Autodesk Fusion 360 part; units mm, degrees
(part 2 of 2)
  spline S18 degree 5 poles (-7.2517, 9.4747) (-7.3168, 9.512) (-7.4501, 9.5899) (-7.66, 9.7166) (-7.9595, 9.9067) (-8.358, 10.1768) (-8.767, 10.4716) (-9.1708, 10.7803) (-9.5541, 11.0901) (-9.9048, 11.3876) (-10.2171, 11.6603) (-10.4929, 11.8976) (-10.7391, 12.0922) (-10.9658, 12.2407) (-11.1836, 12.3449) (-11.4019, 12.4133) (-11.6267, 12.4594) (-11.861, 12.4958) (-12.1043, 12.5285) (-12.3522, 12.5507) (-12.5988, 12.5473) (-12.8401, 12.5021) (-13.0767, 12.404) (-13.3168, 12.2526) (-13.5718, 12.0543) (-13.8538, 11.8189) (-14.1722, 11.5576) (-14.5304, 11.2787) (-14.9249, 10.987) (-15.3481, 10.6852) (-15.7889, 10.3744) (-16.2353, 10.0552) (-16.6753, 9.7283) (-17.0991, 9.3955) (-17.5005, 9.0606) (-17.8781, 8.73) (-18.2334, 8.4108) (-18.5695, 8.11) (-18.8894, 7.8327) (-19.1946, 7.5816) (-19.4837, 7.3549) (-19.7507, 7.1453) (-19.9856, 6.9408) (-20.1783, 6.7275) (-20.3206, 6.4921) (-20.41, 6.2244) (-20.4512, 5.9192) (-20.4542, 5.5754) (-20.432, 5.194) (-20.3978, 4.777) (-20.3627, 4.3258) (-20.3339, 3.8398) (-20.3149, 3.3177) (-20.3063, 2.7575) (-20.3067, 2.1576) (-20.3131, 1.5176) (-20.3215, 0.8388) (-20.3279, 0.1251) (-20.3285, -0.6164) (-20.3207, -1.3746) (-20.3034, -2.1349) (-20.2759, -2.8807) (-20.239, -3.5949) (-20.1938, -4.2607) (-20.1419, -4.8634) (-20.0857, -5.3913) (-20.0274, -5.8373) (-19.9695, -6.1998) (-19.9146, -6.4846) (-19.8639, -6.7043) (-19.814, -6.8757) (-19.7546, -7.0182) (-19.6644, -7.1514) (-19.5198, -7.2925) (-19.3074, -7.4536) (-19.0351, -7.6386) (-18.7247, -7.8455) (-18.4043, -8.0673) (-18.1006, -8.2943) (-17.8313, -8.5156) (-17.5973, -8.7207) (-17.3875, -8.9016) (-17.1846, -9.0544) (-16.9699, -9.1809) (-16.7295, -9.2913) (-16.4555, -9.402) (-16.1448, -9.531) (-15.7988, -9.6939) (-15.4216, -9.8999) (-15.0203, -10.1472) (-14.604, -10.4266) (-14.1834, -10.7236) (-13.7708, -11.0211) (-13.3794, -11.3028) (-13.023, -11.5549) (-12.7157, -11.7699) (-12.4712, -11.9479) (-12.2956, -12.0935) (-12.1833, -12.2134) (-12.1094, -12.313) (-12.0269, -12.3943) (-11.8938, -12.4605) (-11.7016, -12.5203) (-11.4667, -12.5825) (-11.2156, -12.6491) (-10.971, -12.7069) (-10.7469, -12.7327) (-10.5487, -12.7034) (-10.3698, -12.6053) (-10.1927, -12.4403) (-9.9959, -12.2196) (-9.76, -11.9595) (-9.4757, -11.6758) (-9.1465, -11.3808) (-8.7837, -11.084) (-8.4031, -10.7925) (-8.0218, -10.5104) (-7.6537, -10.2396) (-7.3069, -9.9797) (-6.9789, -9.7282) (-6.6609, -9.4812) (-6.3406, -9.2345) (-6.0056, -8.9846) (-5.6472, -8.7296) (-5.2637, -8.4697) (-4.8637, -8.2089) (-4.4636, -7.9529) (-4.0833, -7.7077) (-3.743, -7.4773) (-3.4589, -7.2624) (-3.2401, -7.0583) (-3.084, -6.8528) (-2.9785, -6.6295) (-2.9084, -6.3746) (-2.8592, -6.0822) (-2.8238, -5.7618) (-2.801, -5.4333) (-2.7922, -5.1182) (-2.7991, -4.8328) (-2.8206, -4.5793) (-2.8513, -4.3413) (-2.8836, -4.0939) (-2.9103, -3.8111) (-2.9266, -3.4759) (-2.9318, -3.0849) (-2.9277, -2.6437) (-2.9179, -2.1642) (-2.9066, -1.6617) (-2.898, -1.1512) (-2.8953, -0.6444) (-2.8997, -0.1471) (-2.9108, 0.3397) (-2.9278, 0.8181) (-2.9493, 1.2924) (-2.9742, 1.7676) (-3.0021, 2.2478) (-3.0339, 2.7355) (-3.0722, 3.2296) (-3.12, 3.7267) (-3.1797, 4.2204) (-3.2516, 4.7025) (-3.3331, 5.1626) (-3.4174, 5.5887) (-3.4923, 5.9676) (-3.54, 6.2851) (-3.5462, 6.5321) (-3.5083, 6.7085) (-3.4435, 6.8282) (-3.397, 6.9241) (-3.4176, 7.0322) (-3.5281, 7.1723) (-3.7286, 7.3497) (-4.0048, 7.5599) (-4.3366, 7.7927) (-4.7008, 8.035) (-5.0747, 8.2729) (-5.4384, 8.494) (-5.7777, 8.6901) (-6.0873, 8.859) (-6.3735, 9.0076) (-6.6504, 9.1484) (-6.8781, 9.2669) (-7.0596, 9.3657) (-7.1866, 9.4373) (-7.2517, 9.4747) knots 0 0 0 0 0 0 0.00555556 0.01111111 0.01666667 0.02222222 0.02777778 0.03333333 0.03888889 0.04444444 0.05 0.05555556 0.06111111 0.06666667 0.07222222 0.07777778 0.08333333 0.08888889 0.09444444 0.1 0.10555556 0.11111111 0.11666667 0.12222222 0.12777778 0.13333333 0.13888889 0.14444444 0.15 0.15555556 0.16111111 0.16666667 0.17222222 0.17777778 0.18333333 0.18888889 0.19444444 0.2 0.20555556 0.21111111 0.21666667 0.22222222 0.22777778 0.23333333 0.23888889 0.24444444 0.25 0.25555556 0.26111111 0.26666667 0.27222222 0.27777778 0.28333333 0.28888889 0.29444444 0.3 0.30555556 0.31111111 0.31666667 0.32222222 0.32777778 0.33333333 0.33888889 0.34444444 0.35 0.35555556 0.36111111 0.36666667 0.37222222 0.37777778 0.38333333 0.38888889 0.39444444 0.4 0.40555556 0.41111111 0.41666667 0.42222222 0.42777778 0.43333333 0.43888889 0.44444444 0.45 0.45555556 0.46111111 0.46666667 0.47222222 0.47777778 0.48333333 0.48888889 0.49444444 0.5 0.50555556 0.51111111 0.51666667 0.52222222 0.52777778 0.53333333 0.53888889 0.54444444 0.55 0.55555556 0.56111111 0.56666667 0.57222222 0.57777778 0.58333333 0.58888889 0.59444444 0.6 0.60555556 0.61111111 0.61666667 0.62222222 0.62777778 0.63333333 0.63888889 0.64444444 0.65 0.65555556 0.66111111 0.66666667 0.67222222 0.67777778 0.68333333 0.68888889 0.69444444 0.7 0.70555556 0.71111111 0.71666667 0.72222222 0.72777778 0.73333333 0.73888889 0.74444444 0.75 0.75555556 0.76111111 0.76666667 0.77222222 0.77777778 0.78333333 0.78888889 0.79444444 0.8 0.80555556 0.81111111 0.81666667 0.82222222 0.82777778 0.83333333 0.83888889 0.84444444 0.85 0.85555556 0.86111111 0.86666667 0.87222222 0.87777778 0.88333333 0.88888889 0.89444444 0.9 0.90555556 0.91111111 0.91666667 0.92222222 0.92777778 0.93333333 0.93888889 0.94444444 0.95 0.95555556 0.96111111 0.96666667 0.97222222 0.97777778 0.98333333 0.98888889 0.99444444 1 1 1 1 1 1
  spline S19 degree 5 poles (-40.2, 19.4351) (-40.1495, 19.476) (-40.0504, 19.5572) (-39.9066, 19.6793) (-39.7159, 19.8475) (-39.453, 20.0809) (-39.14, 20.3488) (-38.758, 20.6585) (-38.3003, 21.011) (-37.7793, 21.3986) (-37.2214, 21.8068) (-36.6606, 22.217) (-36.1323, 22.6084) (-35.6682, 22.9604) (-35.2892, 23.2551) (-35.0009, 23.4794) (-34.785, 23.6273) (-34.6008, 23.7015) (-34.4066, 23.7119) (-34.1775, 23.6741) (-33.9251, 23.6084) (-33.6789, 23.5323) (-33.471, 23.4545) (-33.3152, 23.365) (-33.2061, 23.2403) (-33.1308, 23.057) (-33.0779, 22.8053) (-33.0386, 22.4862) (-33.0065, 22.1076) (-32.977, 21.6793) (-32.9478, 21.209) (-32.9178, 20.7018) (-32.8874, 20.1618) (-32.8573, 19.593) (-32.8288, 19.0006) (-32.8028, 18.3916) (-32.7799, 17.7766) (-32.7595, 17.1703) (-32.7405, 16.59) (-32.7226, 16.0527) (-32.7068, 15.5729) (-32.6961, 15.1596) (-32.6968, 14.8144) (-32.7192, 14.5282) (-32.7779, 14.2806) (-32.8886, 14.0459) (-33.0655, 13.7986) (-33.3183, 13.5197) (-33.6503, 13.1997) (-34.0603, 12.8358) (-34.5422, 12.4316) (-35.0857, 11.9949) (-35.6774, 11.5367) (-36.3007, 11.0697) (-36.9368, 10.6072) (-37.5651, 10.161) (-38.1648, 9.7421) (-38.7171, 9.3602) (-39.207, 9.0239) (-39.6256, 8.7411) (-39.9715, 8.5185) (-40.2533, 8.362) (-40.4915, 8.2769) (-40.7195, 8.2675) (-40.9724, 8.3353) (-41.2796, 8.4772) (-41.6523, 8.6835) (-42.0841, 8.9384) (-42.5573, 9.2226) (-43.047, 9.5149) (-43.5268, 9.7948) (-43.9737, 10.0443) (-44.373, 10.25) (-44.7229, 10.4053) (-45.0277, 10.511) (-45.2924, 10.5774) (-45.5183, 10.6236) (-45.6944, 10.6818) (-45.8041, 10.7888) (-45.8443, 10.969) (-45.8452, 11.2162) (-45.854, 11.5036) (-45.9111, 11.7986) (-46.0261, 12.078) (-46.1667, 12.3364) (-46.2851, 12.578) (-46.3335, 12.8126) (-46.2887, 13.0483) (-46.157, 13.2899) (-45.9588, 13.5405) (-45.7197, 13.8029) (-45.4577, 14.0807) (-45.1827, 14.3782) (-44.899, 14.6991) (-44.6065, 15.0456) (-44.3031, 15.4178) (-43.9864, 15.8126) (-43.6548, 16.2231) (-43.3079, 16.6403) (-42.9465, 17.0538) (-42.5731, 17.4534) (-42.1923, 17.8296) (-41.8102, 18.1754) (-41.4361, 18.4869) (-41.0804, 18.7639) (-40.7523, 19.0098) (-40.5162, 19.1867) (-40.3537, 19.3122) (-40.2505, 19.3943) (-40.2, 19.4351) knots 0 0 0 0 0 0 0.00952381 0.01904762 0.02857143 0.03809524 0.04761905 0.05714286 0.06666667 0.07619048 0.08571429 0.0952381 0.1047619 0.11428571 0.12380952 0.13333333 0.14285714 0.15238095 0.16190476 0.17142857 0.18095238 0.19047619 0.2 0.20952381 0.21904762 0.22857143 0.23809524 0.24761905 0.25714286 0.26666667 0.27619048 0.28571429 0.2952381 0.3047619 0.31428571 0.32380952 0.33333333 0.34285714 0.35238095 0.36190476 0.37142857 0.38095238 0.39047619 0.4 0.40952381 0.41904762 0.42857143 0.43809524 0.44761905 0.45714286 0.46666667 0.47619048 0.48571429 0.4952381 0.5047619 0.51428571 0.52380952 0.53333333 0.54285714 0.55238095 0.56190476 0.57142857 0.58095238 0.59047619 0.6 0.60952381 0.61904762 0.62857143 0.63809524 0.64761905 0.65714286 0.66666667 0.67619048 0.68571429 0.6952381 0.7047619 0.71428571 0.72380952 0.73333333 0.74285714 0.75238095 0.76190476 0.77142857 0.78095238 0.79047619 0.8 0.80952381 0.81904762 0.82857143 0.83809524 0.84761905 0.85714286 0.86666667 0.87619048 0.88571429 0.8952381 0.9047619 0.91428571 0.92380952 0.93333333 0.94285714 0.95238095 0.96190476 0.97142857 0.98095238 0.99047619 1 1 1 1 1 1
  spline S20 degree 5 poles (-25.9, 8.6722) (-25.985, 8.7472) (-26.1636, 8.9038) (-26.4606, 9.1593) (-26.9174, 9.5357) (-27.5668, 10.0317) (-28.2524, 10.5092) (-28.9256, 10.925) (-29.5423, 11.2473) (-30.0755, 11.4668) (-30.5261, 11.6065) (-30.9112, 11.7) (-31.2555, 11.7738) (-31.5798, 11.825) (-31.895, 11.8119) (-32.2111, 11.6854) (-32.5455, 11.4204) (-32.9254, 11.0283) (-33.3782, 10.5415) (-33.9245, 10.003) (-34.5714, 9.4557) (-35.3028, 8.9294) (-36.0811, 8.4376) (-36.8574, 7.9821) (-37.5787, 7.5557) (-38.1966, 7.1453) (-38.6754, 6.7349) (-39.0006, 6.3087) (-39.1866, 5.8539) (-39.2658, 5.3609) (-39.2789, 4.8233) (-39.2645, 4.2377) (-39.2483, 3.604) (-39.2441, 2.9246) (-39.2565, 2.2046) (-39.2832, 1.4506) (-39.3166, 0.6707) (-39.3466, -0.1262) (-39.3626, -0.9307) (-39.3551, -1.7331) (-39.3175, -2.5235) (-39.2478, -3.2923) (-39.1505, -4.0305) (-39.0386, -4.7293) (-38.934, -5.3811) (-38.859, -5.9806) (-38.8263, -6.5264) (-38.8314, -7.0222) (-38.8419, -7.4784) (-38.7927, -7.9128) (-38.6115, -8.3453) (-38.2383, -8.7928) (-37.6502, -9.2644) (-36.8736, -9.7584) (-35.9659, -10.2657) (-35.0038, -10.7727) (-34.0691, -11.2633) (-33.2357, -11.7224) (-32.5556, -12.138) (-32.0455, -12.504) (-31.6741, -12.823) (-31.3816, -13.0981) (-31.0981, -13.3257) (-30.7625, -13.488) (-30.3407, -13.5461) (-29.8195, -13.456) (-29.202, -13.1834) (-28.5022, -12.7205) (-27.7405, -12.0969) (-26.9418, -11.3666) (-26.1335, -10.5978) (-25.3437, -9.8614) (-24.599, -9.2207) (-23.9227, -8.7192) (-23.3325, -8.3717) (-22.8388, -8.1491) (-22.4442, -7.9856) (-22.1471, -7.8007) (-21.9423, -7.5148) (-21.8245, -7.0705) (-21.7873, -6.4359) (-21.8233, -5.6001) (-21.9228, -4.5723) (-22.0736, -3.3784) (-22.26, -2.0594) (-22.4625, -0.6688) (-22.6569, 0.7295) (-22.8183, 2.0679) (-22.9253, 3.2821) (-22.9644, 4.3176) (-22.9339, 5.137) (-22.8485, 5.7265) (-22.743, 6.1028) (-22.6769, 6.3201) (-22.7387, 6.4772) (-22.9915, 6.6663) (-23.409, 6.9138) (-23.9101, 7.2016) (-24.4022, 7.495) (-24.8205, 7.7682) (-25.1705, 8.0316) (-25.4353, 8.2591) (-25.6538, 8.454) (-25.815, 8.5972) (-25.9, 8.6722) knots 0 0 0 0 0 0 0.01 0.02 0.03 0.04 0.05 0.06 0.07 0.08 0.09 0.1 0.11 0.12 0.13 0.14 0.15 0.16 0.17 0.18 0.19 0.2 0.21 0.22 0.23 0.24 0.25 0.26 0.27 0.28 0.29 0.3 0.31 0.32 0.33 0.34 0.35 0.36 0.37 0.38 0.39 0.4 0.41 0.42 0.43 0.44 0.45 0.46 0.47 0.48 0.49 0.5 0.51 0.52 0.53 0.54 0.55 0.56 0.57 0.58 0.59 0.6 0.61 0.62 0.63 0.64 0.65 0.66 0.67 0.68 0.69 0.7 0.71 0.72 0.73 0.74 0.75 0.76 0.77 0.78 0.79 0.8 0.81 0.82 0.83 0.84 0.85 0.86 0.87 0.88 0.89 0.9 0.91 0.92 0.93 0.94 0.95 0.96 0.97 0.98 0.99 1 1 1 1 1 1
  spline S21 degree 5 poles (-40.2, -20.1) (-40.0706, -20.2092) (-39.8095, -20.4267) (-39.4106, -20.7506) (-38.8646, -21.1776) (-38.1588, -21.703) (-37.4319, -22.2187) (-36.6888, -22.7225) (-35.9379, -23.2109) (-35.1929, -23.6784) (-34.4731, -24.1178) (-33.8055, -24.5194) (-33.2254, -24.8707) (-32.767, -25.1588) (-32.4534, -25.373) (-32.2867, -25.5066) (-32.2382, -25.5597) (-32.2349, -25.5425) (-32.1855, -25.4699) (-32.0198, -25.3543) (-31.7004, -25.2031) (-31.3079, -25.0569) (-30.9345, -24.9337) (-30.6507, -24.8456) (-30.5, -24.8) knots 0 0 0 0 0 0 0.05 0.1 0.15 0.2 0.25 0.3 0.35 0.4 0.45 0.5 0.55 0.6 0.65 0.7 0.75 0.8 0.85 0.9 0.95 1 1 1 1 1 1
  spline S22 degree 5 poles (-30.5, -24.8) (-30.4964, -24.8106) (-30.4893, -24.8249) (-30.4795, -24.8259) (-30.4679, -24.7865) (-30.4563, -24.6722) (-30.4484, -24.5015) (-30.4456, -24.2861) (-30.4488, -24.0388) (-30.4584, -23.7715) (-30.4736, -23.4928) (-30.4933, -23.2086) (-30.5154, -22.9229) (-30.538, -22.6377) (-30.5591, -22.3537) (-30.5769, -22.0706) (-30.5902, -21.7877) (-30.5984, -21.5037) (-30.6017, -21.2168) (-30.6011, -20.925) (-30.5987, -20.6258) (-30.5975, -20.317) (-30.6016, -19.9961) (-30.6152, -19.6614) (-30.6417, -19.3126) (-30.6835, -18.9504) (-30.7409, -18.5781) (-30.8118, -18.2012) (-30.8907, -17.8283) (-30.97, -17.47) (-31.042, -17.1373) (-31.0999, -16.8407) (-31.1399, -16.5885) (-31.1622, -16.3858) (-31.1736, -16.2329) (-31.1863, -16.1249) (-31.214, -16.0519) (-31.2687, -15.9993) (-31.3575, -15.949) (-31.4842, -15.883) (-31.6493, -15.7887) (-31.8513, -15.6612) (-32.0873, -15.5007) (-32.3533, -15.3116) (-32.6447, -15.1001) (-32.9573, -14.8733) (-33.2878, -14.6368) (-33.6334, -14.3946) (-33.992, -14.1497) (-34.3617, -13.904) (-34.7407, -13.6587) (-35.1266, -13.4147) (-35.5167, -13.1729) (-35.9073, -12.9341) (-36.2936, -12.6997) (-36.6695, -12.4717) (-37.0284, -12.2525) (-37.3639, -12.0448) (-37.6698, -11.8513) (-37.9417, -11.6746) (-38.1766, -11.517) (-38.3742, -11.3804) (-38.537, -11.2662) (-38.6707, -11.1747) (-38.7834, -11.1053) (-38.8853, -11.0562) (-38.9886, -11.0241) (-39.1062, -11.0048) (-39.2492, -10.9943) (-39.4255, -10.9898) (-39.6398, -10.9896) (-39.8434, -10.9922) (-40.0145, -10.9955) (-40.1368, -10.9984) (-40.2, -11) knots 0 0 0 0 0 0 0.01428571 0.02857143 0.04285714 0.05714286 0.07142857 0.08571429 0.1 0.11428571 0.12857143 0.14285714 0.15714286 0.17142857 0.18571429 0.2 0.21428571 0.22857143 0.24285714 0.25714286 0.27142857 0.28571429 0.3 0.31428571 0.32857143 0.34285714 0.35714286 0.37142857 0.38571429 0.4 0.41428571 0.42857143 0.44285714 0.45714286 0.47142857 0.48571429 0.5 0.51428571 0.52857143 0.54285714 0.55714286 0.57142857 0.58571429 0.6 0.61428571 0.62857143 0.64285714 0.65714286 0.67142857 0.68571429 0.7 0.71428571 0.72857143 0.74285714 0.75714286 0.77142857 0.78571429 0.8 0.81428571 0.82857143 0.84285714 0.85714286 0.87142857 0.88571429 0.9 0.91428571 0.92857143 0.94285714 0.95714286 0.97142857 0.98571429 1 1 1 1 1 1
  spline S23 degree 5 poles (-11.3807, -26) (-11.3882, -25.9105) (-11.4027, -25.7292) (-11.4225, -25.45) (-11.4453, -25.0635) (-11.4676, -24.5565) (-11.484, -24.0265) (-11.4948, -23.4746) (-11.5006, -22.903) (-11.5022, -22.315) (-11.501, -21.7149) (-11.4985, -21.1088) (-11.4968, -20.5044) (-11.4986, -19.911) (-11.506, -19.3381) (-11.5212, -18.7953) (-11.5452, -18.2908) (-11.5783, -17.8313) (-11.619, -17.4208) (-11.6644, -17.0598) (-11.7089, -16.7448) (-11.7463, -16.4683) (-11.7735, -16.2221) (-11.7943, -15.999) (-11.8223, -15.795) (-11.8853, -15.6121) (-12.009, -15.4539) (-12.2023, -15.3221) (-12.4367, -15.2119) (-12.6554, -15.113) (-12.8073, -15.0148) (-12.8724, -14.9108) (-12.8948, -14.8037) (-12.9486, -14.6996) (-13.0853, -14.5989) (-13.3163, -14.4937) (-13.6305, -14.3727) (-14.0028, -14.2244) (-14.4069, -14.0412) (-14.8248, -13.8219) (-15.2451, -13.5706) (-15.6619, -13.2949) (-16.0729, -13.0046) (-16.4785, -12.71) (-16.8799, -12.4202) (-17.2784, -12.1423) (-17.6731, -11.879) (-18.0611, -11.629) (-18.4373, -11.3894) (-18.7951, -11.1568) (-19.1266, -10.9294) (-19.4222, -10.7085) (-19.6719, -10.4999) (-19.8642, -10.3165) (-19.9921, -10.1728) (-20.0597, -10.0773) (-20.0887, -10.0256) (-20.1237, -9.9948) (-20.2069, -9.9655) (-20.3606, -9.9346) (-20.5879, -9.9046) (-20.8677, -9.8779) (-21.1654, -9.856) (-21.4457, -9.842) (-21.6827, -9.8418) (-21.8755, -9.8663) (-22.048, -9.9302) (-22.2323, -10.0471) (-22.4581, -10.2255) (-22.7378, -10.4644) (-23.0703, -10.7553) (-23.4448, -11.0849) (-23.8443, -11.4371) (-24.2493, -11.7957) (-24.642, -12.1464) (-25.0092, -12.4795) (-25.3469, -12.7922) (-25.6587, -13.0874) (-25.9525, -13.3714) (-26.2386, -13.6516) (-26.5268, -13.9345) (-26.8236, -14.2239) (-27.1301, -14.5183) (-27.4395, -14.8093) (-27.7397, -15.0856) (-28.0164, -15.336) (-28.2555, -15.5537) (-28.4458, -15.7392) (-28.5816, -15.9048) (-28.6652, -16.076) (-28.7033, -16.2816) (-28.7055, -16.5469) (-28.6814, -16.8826) (-28.6397, -17.2845) (-28.5884, -17.7384) (-28.5342, -18.2242) (-28.483, -18.7198) (-28.4394, -19.2053) (-28.4066, -19.6669) (-28.3867, -20.1014) (-28.3802, -20.5139) (-28.3864, -20.9144) (-28.4038, -21.3151) (-28.4297, -21.727) (-28.4606, -22.1572) (-28.4923, -22.6051) (-28.5201, -23.0611) (-28.5393, -23.5103) (-28.5459, -23.9357) (-28.5369, -24.3208) (-28.511, -24.6538) (-28.4693, -24.9298) (-28.4156, -25.1551) (-28.3556, -25.3436) (-28.2954, -25.5118) (-28.2397, -25.6733) (-28.2007, -25.8027) (-28.1749, -25.9009) (-28.1593, -25.9669) (-28.1519, -26) knots 0 0 0 0 0 0 0.00869565 0.0173913 0.02608696 0.03478261 0.04347826 0.05217391 0.06086957 0.06956522 0.07826087 0.08695652 0.09565217 0.10434783 0.11304348 0.12173913 0.13043478 0.13913043 0.14782609 0.15652174 0.16521739 0.17391304 0.1826087 0.19130435 0.2 0.20869565 0.2173913 0.22608696 0.23478261 0.24347826 0.25217391 0.26086957 0.26956522 0.27826087 0.28695652 0.29565217 0.30434783 0.31304348 0.32173913 0.33043478 0.33913043 0.34782609 0.35652174 0.36521739 0.37391304 0.3826087 0.39130435 0.4 0.40869565 0.4173913 0.42608696 0.43478261 0.44347826 0.45217391 0.46086957 0.46956522 0.47826087 0.48695652 0.49565217 0.50434783 0.51304348 0.52173913 0.53043478 0.53913043 0.54782609 0.55652174 0.56521739 0.57391304 0.5826087 0.59130435 0.6 0.60869565 0.6173913 0.62608696 0.63478261 0.64347826 0.65217391 0.66086957 0.66956522 0.67826087 0.68695652 0.69565217 0.70434783 0.71304348 0.72173913 0.73043478 0.73913043 0.74782609 0.75652174 0.76521739 0.77391304 0.7826087 0.79130435 0.8 0.80869565 0.8173913 0.82608696 0.83478261 0.84347826 0.85217391 0.86086957 0.86956522 0.87826087 0.88695652 0.89565217 0.90434783 0.91304348 0.92173913 0.93043478 0.93913043 0.94782609 0.95652174 0.96521739 0.97391304 0.9826087 0.99130435 1 1 1 1 1 1
  spline S24 degree 5 poles (-35.5, -26) (-35.5833, -25.9533) (-35.751, -25.8583) (-36.0053, -25.7111) (-36.3502, -25.5056) (-36.7917, -25.2319) (-37.2442, -24.9401) (-37.7088, -24.629) (-38.1855, -24.2981) (-38.6736, -23.9487) (-39.1723, -23.5822) (-39.5789, -23.2765) (-39.8879, -23.0408) (-40.0957, -22.8807) (-40.2, -22.8) knots 0 0 0 0 0 0 0.1 0.2 0.3 0.4 0.5 0.6 0.7 0.8 0.9 1 1 1 1 1 1
  spline S25 degree 5 poles (14.0457, 25.2) (14.0267, 25.2099) (13.9912, 25.2275) (13.9457, 25.2475) (13.8992, 25.2627) (13.862, 25.2643) (13.8508, 25.2507) (13.8556, 25.2299) (13.8653, 25.2109) (13.8718, 25.2) knots 0 0 0 0 0 0 0.2 0.4 0.6 0.8 1 1 1 1 1 1
  line L8 (14.1082, 25.1676) -> (13.9832, 25.2324)
  line L9 (13.8589, 25.2215) -> (13.8846, 25.1785)
  spline S26 degree 5 poles (21.4, 18.8332) (21.4048, 18.832) (21.414, 18.8302) (21.426, 18.8289) (21.4384, 18.8303) (21.4449, 18.8396) (21.4384, 18.8571) (21.4237, 18.8786) (21.4087, 18.8973) (21.4, 18.9077) knots 0 0 0 0 0 0 0.2 0.4 0.6 0.8 1 1 1 1 1 1
  line L10 (21.44, 18.8599) -> (21.36, 18.9555)
  spline S27 degree 5 poles (21.4, 18.75) (21.3631, 18.7928) (21.2889, 18.8779) (21.1763, 19.0041) (21.0237, 19.1697) (20.829, 19.3722) (20.6305, 19.5711) (20.4291, 19.7678) (20.2261, 19.9649) (20.0229, 20.1657) (19.82, 20.3737) (19.6162, 20.5922) (19.408, 20.8236) (19.1896, 21.0695) (18.9547, 21.3303) (18.6977, 21.6059) (18.4144, 21.8949) (18.1039, 22.1949) (17.7674, 22.5031) (17.4075, 22.8161) (17.0278, 23.1307) (16.6321, 23.4439) (16.2236, 23.7531) (15.8046, 24.0568) (15.3767, 24.3539) (14.9409, 24.6439) (14.5864, 24.87) (14.3173, 25.0363) (14.1365, 25.1457) (14.0457, 25.2) knots 0 0 0 0 0 0 0.04 0.08 0.12 0.16 0.2 0.24 0.28 0.32 0.36 0.4 0.44 0.48 0.52 0.56 0.6 0.64 0.68 0.72 0.76 0.8 0.84 0.88 0.92 0.96 1 1 1 1 1 1
  line L11 (-40.2, -0.0059) -> (-9.4, -0.0059) construction
  line L12 (-9.4, -0.0059) -> (4.6, -0.0059) construction
  line L13 (-9.4, -0.0059) -> (-23.4, -0.0059) construction
  line L14 (4.6, -0.0059) -> (4.6, -6.0059) construction
  line L15 (-23.4, -0.0059) -> (-23.4, 5.9941) construction
  line L16 (19.4, -22) -> (19.4, 21.2)
  line L17 (17.4, 23.2) -> (-36.2, 23.2)
  line L18 (-38.2, 21.2) -> (-38.2, -22)
  line L19 (-36.2, -24) -> (17.4, -24)
  arc A23 (17.4, -24) -> (19.4, -22) centre (17.4, -22) ccw
  arc A24 (19.4, 21.2) -> (17.4, 23.2) centre (17.4, 21.2) ccw
  arc A25 (-36.2, 23.2) -> (-38.2, 21.2) centre (-36.2, 21.2) ccw
  arc A26 (-38.2, -22) -> (-36.2, -24) centre (-36.2, -22) ccw
  line L20 (4.6, -6.0059) -> (4.6, -8.2559)
  line L21 (-21.475, 9.1404) -> (2.675, 9.1404)
  line L22 (2.675, 9.1404) -> (2.675, -9.1523)
  line L23 (2.675, -9.1523) -> (-21.475, -9.1523)
  line L24 (-21.475, -9.1523) -> (-21.475, 9.1404)
  line L25 (-21.475, 9.1404) -> (2.675, -9.1523) construction
  line L26 (2.675, 9.1404) -> (-21.475, -9.1523) construction
  line L27 (-22.475, 10.1404) -> (3.675, 10.1404)
  line L28 (3.675, 10.1404) -> (3.675, -10.1523)
  line L29 (3.675, -10.1523) -> (-22.475, -10.1523)
  line L30 (-22.475, -10.1523) -> (-22.475, 10.1404)
  line L31 (2.675, 9.1404) -> (-21.475, 9.1404) construction
  line L32 (-21.475, 9.1404) -> (-21.475, -8.6556) construction
  line L33 (-21.475, -8.6556) -> (2.675, -8.6556) construction
  line L34 (2.675, -8.6556) -> (2.675, 9.1404) construction
  point P0 (7.051, -15.0762)
  point P1 (6.8334, -14.8314)
  point P2 (5.8, -14)
  point P3 (5.004, -13.2468)
  point P4 (3, -11.9)
  point P5 (2.1938, -11.2552)
  point P6 (0.6849, -10.1414)
  point P7 (-0.5285, -9.419)
  point P8 (-1.3037, -9.3762)
  point P9 (-2.3649, -9.4289)
  point P10 (-2.8331, -9.5374)
  point P11 (-5.5, -11.6)
  point P12 (-8.6, -14.2)
  point P13 (-9.7727, -15.2896)
  point P14 (-9.8476, -15.4656)
  point P15 (-9.85, -15.9)
  point P16 (-9.9, -19.4)
  point P17 (-9.7, -24)
  point P18 (19.8, -9.5)
  point P19 (18.3, -8.5)
  point P20 (18, -8.4)
  point P21 (16.7, -8.45)
  point P22 (16.2684, -8.4722)
  point P23 (16.0731, -8.5685)
  point P24 (13.8, -10.4)
  point P25 (10.9, -12.8)
  point P26 (9.4, -14.3)
  point P27 (19.1566, -6.6508)
  point P28 (18.8, -6.4)
  point P29 (18.7, -6.3)
  point P30 (18.55, -5.75)
  point P31 (18.2, -4.9)
  point P32 (18.3, -3.5)
  point P33 (18.5, -1.9)
  point P34 (18.5, 1.2)
  point P35 (18.3, 5.1)
  point P36 (18.3, 6.4)
  point P37 (18.1, 7.7)
  point P38 (18.1, 7.9)
  point P39 (18.9, 8.7)
  point P40 (19.8, 9.4)
  point P41 (13.5, -6.7)
  point P42 (11.8, -8.2)
  point P43 (11.2358, -8.9708)
  point P44 (9.7, -10.7)
  point P45 (8.9, -11.5)
  point P46 (7.1, -11.8)
  point P47 (6.9515, -11.7173)
  point P48 (6.7172, -11.5441)
  point P49 (6.1776, -11.2025)
  point P50 (5.2568, -10.5309)
  point P51 (3.2, -9)
  point P52 (1.1, -7.7)
  point P53 (-0.3, -6.9)
  point P54 (-0.4238, -6.8342)
  point P55 (-0.5, -6.65)
  point P56 (-1.1, -5.6)
  point P57 (-1.03, -5.44)
  point P58 (-1, -5.06)
  point P59 (-1.2, 0.8)
  point P60 (-1.4, 3.6)
  point P61 (-1.3471, 6.431)
  point P62 (-1.25, 6.6)
  point P63 (-0.95, 7)
  point P64 (0.1, 8.2)
  point P65 (1.3456, 9.4747)
  point P66 (2.8, 10.4)
  point P67 (4.9, 11.6)
  point P68 (6.3872, 12.6401)
  point P69 (6.6424, 12.7645)
  point P70 (6.8339, 12.9272)
  point P71 (6.853, 13.1666)
  point P72 (8.7389, 12.6752)
  point P73 (9.9, 11.8)
  point P74 (11.8532, 10.4191)
  point P75 (14.6, 8.6)
  point P76 (15.0195, 8.3059)
  point P77 (15.3239, 7.4349)
  point P78 (15.4241, 7.0187)
  point P79 (15.46, 6.97)
  point P80 (15.47, 6.82)
  point P81 (15.5, 5.3)
  point P82 (15.7, 1.7)
  point P83 (15.9, -1.6)
  point P84 (16, -4.7)
  point P85 (19, 12.5)
  point P86 (17.1, 10.8)
  point P87 (16.9413, 10.7222)
  point P88 (15.4242, 10.653)
  point P89 (15.2561, 10.5355)
  point P90 (14.7, 10.9)
  point P91 (13, 12.2)
  point P92 (9.9, 14.1)
  point P93 (8.3, 15.2)
  point P94 (8.1, 15.6)
  point P95 (7.6, 16.4)
  point P96 (7.5842, 24.746)
  point P97 (7.7, 25)
  point P98 (11.1, 24.8)
  point P99 (13.2, 23.5)
  point P100 (15.3, 21.9)
  point P101 (19.7684, 17.8233)
  point P102 (-1.7373, 10.1137)
  point P103 (-2, 10)
  point P104 (-3.9745, 10.1787)
  point P105 (-4.5, 10.5)
  point P106 (-8.6013, 13.0644)
  point P107 (-11, 15)
  point P108 (-11.4088, 17.8233)
  point P109 (-11.8416, 24.856)
  point P110 (-11.8416, 28.1549)
  point P111 (5.5887, 19.6873)
  point P112 (-13.7842, 19.4469)
  point P113 (-13.4708, 14.953)
  point P114 (-14.3, 14.3)
  point P115 (-17.1, 12.1)
  point P116 (-20.1, 9.7)
  point P117 (-20.4418, 9.3773)
  point P118 (-20.9233, 9.2608)
  point P119 (-22.6453, 9.1404)
  point P120 (-23.25, 9.6)
  point P121 (-25.9, 11.2)
  point P122 (-27, 12)
  point P123 (-29.5, 13.6)
  point P124 (-29.7216, 13.8493)
  point P125 (-30.059, 14.4103)
  point P126 (-30.2, 14.8)
  point P127 (-30.275, 15.4915)
  point P128 (-30.5, 18)
  point P129 (-30.6157, 22.6489)
  point P130 (-30.3715, 24.2766)
  point P131 (-37.4, 24)
  point P132 (-9.8, 11.3)
  point P133 (-11.1, 12.3)
  point P134 (-11.9, 12.5)
  point P135 (-12.8, 12.5)
  point P136 (-14, 11.7)
  point P137 (-16.9943, 9.4747)
  point P138 (-19.3, 7.5)
  point P139 (-20.3, 6.5)
  point P140 (-20.4, 4.8)
  point P141 (-20.3271, -0.0959)
  point P142 (-20, -6)
  point P143 (-19.8, -6.9)
  point P144 (-19.5, -7.3)
  point P145 (-18.1, -8.3)
  point P146 (-17.1, -9.1)
  point P147 (-15.8, -9.7)
  point P148 (-13.1, -11.5)
  point P149 (-12.2, -12.2)
  point P150 (-12, -12.4)
  point P151 (-11.4, -12.6)
  point P152 (-10.6, -12.7)
  point P153 (-9.8455, -12.0566)
  point P154 (-7.6497, -10.2354)
  point P155 (-5.6, -8.7)
  point P156 (-3.4, -7.2)
  point P157 (-2.9, -6.3)
  point P158 (-2.8, -4.9)
  point P159 (-2.9, -3.9)
  point P160 (-2.9, -1.2)
  point P161 (-3, 2.2)
  point P162 (-3.4, 5.5)
  point P163 (-3.5, 6.7)
  point P164 (-3.4128, 6.9443)
  point P165 (-3.8, 7.4)
  point P166 (-5.8, 8.7)
  point P167 (-38.7, 20.7)
  point P168 (-35.1, 23.4)
  point P169 (-34.4, 23.7)
  point P170 (-33.6, 23.5)
  point P171 (-33.2, 23.2)
  point P172 (-33, 22)
  point P173 (-32.8, 18.3)
  point P174 (-32.7, 14.9)
  point P175 (-33, 13.9)
  point P176 (-36.4, 11)
  point P177 (-40.2, 8.4)
  point P178 (-41.1, 8.4)
  point P179 (-43.9, 10)
  point P180 (-45.4, 10.6)
  point P181 (-45.7987, 10.8317)
  point P182 (-45.9, 11.7)
  point P183 (-46.3, 12.7)
  point P184 (-45.9, 13.6)
  point P185 (-44.4, 15.3)
  point P186 (-42, 18)
  point P187 (-29.4758, 11.2)
  point P188 (-31.171, 11.7528)
  point P189 (-32.0838, 11.7202)
  point P190 (-34.2191, 9.7643)
  point P191 (-38.62, 6.7488)
  point P192 (-39.272, 4.744)
  point P193 (-39.3046, 0.9461)
  point P194 (-39.1579, -3.9438)
  point P195 (-38.8319, -6.9266)
  point P196 (-38.3266, -8.6544)
  point P197 (-32.6217, -12.11)
  point P198 (-31.1, -13.3)
  point P199 (-29.3, -13.2)
  point P200 (-23.7, -8.6)
  point P201 (-22.1, -7.7)
  point P202 (-22.2711, -1.9916)
  point P203 (-22.7504, 6.0736)
  point P204 (-22.8, 6.5)
  point P205 (-24.4, 7.5)
  point P206 (-34.5, -24.1)
  point P207 (-32.3, -25.5)
  point P208 (-32.2, -25.5)
  point P209 (-30.4701, -24.7787)
  point P210 (-30.45, -24.05)
  point P211 (-30.5507, -22.4626)
  point P212 (-30.6, -20.8)
  point P213 (-30.751, -18.538)
  point P214 (-31.1504, -16.4833)
  point P215 (-31.2132, -16.0695)
  point P216 (-31.45, -15.9)
  point P217 (-32.752, -15.0224)
  point P218 (-35.8, -13)
  point P219 (-38.2, -11.5)
  point P220 (-38.8, -11.1)
  point P221 (-39.1501, -11.0031)
  point P222 (-11.5, -21.5)
  point P223 (-11.6407, -17.2566)
  point P224 (-11.7967, -15.9999)
  point P225 (-12.1, -15.4)
  point P226 (-12.8, -15)
  point P227 (-12.9308, -14.7489)
  point P228 (-13.9734, -14.2317)
  point P229 (-17.0471, -12.3049)
  point P230 (-19.4577, -10.6743)
  point P231 (-20.0458, -10.0946)
  point P232 (-20.1193, -10.0045)
  point P233 (-20.41, -9.93)
  point P234 (-21.5633, -9.8444)
  point P235 (-22.253, -10.0699)
  point P236 (-24.7, -12.2)
  point P237 (-26.8, -14.2)
  point P238 (-28.4, -15.7)
  point P239 (-28.7, -16.4)
  point P240 (-28.4374, -19.2586)
  point P241 (-28.453, -22.051)
  point P242 (-28.5, -24.7)
  point P243 (-28.3, -25.5)
  point P244 (-37.6, -24.7)
  point P245 (20.6, 19.6)
  point P246 (19.75, 20.45)
  point P247 (18.7, 21.6)
  point P248 (16.7547, 23.3449)
  point P249 (-9.4, -0.0059)
  dimension "d293" = 1
  dimension "d294" = 1
  dimension "d295" = 30.8
  dimension "d296" = 14
  dimension "d297" = 14
  dimension "d298" = 6
  dimension "d299" = 6
  dimension "d301" = 2
  dimension "d302" = 2.25
  dimension "d304" = -1
  dimension "d356" = 4.2
  text T0 "AGGRC\nTURTLE\nV3.2" font "Arial" height 4.2 align centre top in box 24.1499 x 17.796 at (2.675, 9.1404) x (-1, 0) y (0, -1) spacing 1 kerned
  constraint coincident L2 A4.start
  constraint coincident L3 A4.end
  constraint coincident L3 A6.end
  constraint coincident L2 A8.end
  constraint coincident L2 A9.end
  constraint tangent A5 A11
  constraint tangent A12 A13
  constraint coincident L2 A13.start
  constraint tangent A13 A16
  constraint coincident L2 S0.end
  constraint tangent A5 A17
  constraint tangent A10 A17
  constraint coincident L3 S2.start
  constraint coincident L3 S2.end
  constraint coincident L3 S10.start
  constraint coincident L3 S11.end
  constraint coincident L6 S13.end
  constraint tangent S12 A22
  constraint tangent S13 A22
  constraint coincident L6 S14.start
  constraint coincident L6 S16.end
  constraint coincident L6 S17.start
  constraint coincident L7 S17.end
  constraint coincident L7 S19.start
  constraint coincident L7 P177
  constraint coincident L7 S21.start
  constraint coincident L7 S22.end
  constraint coincident L2 S23.start
  constraint coincident L4 S23.end
  constraint coincident L2 S24.start
  constraint coincident L7 S24.end
  constraint coincident L0 S25.start
  constraint coincident L3 S26.end
  constraint midpoint S25.start L8
  constraint midpoint S25.end L9
  constraint midpoint S26.end L10
  constraint coincident L5 S27.start
  constraint coincident L7 L11.start
  constraint perpendicular L5 L11
  constraint parallel L11 L12
  constraint parallel L11 L13
  constraint perpendicular L12 L14
  constraint perpendicular L13 L15
  constraint tangent L19 A23
  constraint tangent L16 A23
  constraint tangent L16 A24
  constraint tangent L17 A24
  constraint equal A23 A24
  constraint tangent L17 A25
  constraint tangent L18 A25
  constraint equal A23 A25
  constraint tangent L18 A26
  constraint tangent L19 A26
  constraint equal A23 A26
  constraint parallel L14 L20
  constraint horizontal L21
  constraint perpendicular L21 L22
  constraint parallel L21 L23
  constraint parallel L22 L24
  constraint coincident L25 P249
  constraint coincident L26 P249
  constraint coincident P249 L11.end
  constraint coincident L21.start
  constraint coincident S4
  constraint coincident L22
  measures "d293" radius of A17
  measures "d294" radius of A22
  measures "d295" distance of L11.start P249
  measures "d296" distance of P249 L12.end
  measures "d297" distance of P249 L13.end
  measures "d298" distance of L12.end L14.end
  measures "d299" distance of L13.end L15.end
  measures "d301" radius of A23
  measures "d302" distance of L14.end L20.end
extrude "Extrude33" cut sketch "Sketch24" sketch "Sketch24" against normal blind 0.7 contours S27 L16 L17 A24 | S10 S11 L16 L17 | S12 S13 A22 L17 L27 | S2 L16 | S14 S15 S16 L17 L27 L30 | A5 A6 A10 A11 A12 S1 A17 L16 | S18 L27 | S3 S4 S7 S8 S9 L27 L28 | S19 L17 L18 | A4 L16 L19 A23 | S20 L18 L30 | A13 A14 A15 A16 S0 L19 L29 | S18 L29 | S23 L19 L29 | S21 S22 L18 L19 of sketch 2 text T0 bodies 2
chamfer "Chamfer21" distance 1 distance2 1 8 edges at (-7.8958, -25.2, 24.4) (-12.1, -25.2, 15.35) (-7.8958, -25.2, 6.3) (-3.6915, -25.2, 15.35) (-0.4, -25.2, 15.35) (3.8012, -25.2, 24.4) (8.0023, -25.2, 15.35) (3.8012, -25.2, 6.3) measured on face at (28.1341, -25.2, 18.6) measured on face at (28.1341, -25.2, 18.6) measured on face at (28.1341, -25.2, 18.6) measured on face at (28.1341, -25.2, 18.6) measured on face at (28.1341, -25.2, 18.6) measured on face at (28.1341, -25.2, 18.6) measured on face at (28.1341, -25.2, 18.6) measured on face at (28.1341, -25.2, 18.6) tangent chain off on bodies 1
chamfer "Chamfer22" distance 1 distance2 1 4 edges at (28.95, 26, 10.2) (33, 26, 8.25) (28.95, 26, 6.3) (24.9, 26, 8.25) measured on face at (-4.6333, 26, 13.8667) measured on face at (-4.6333, 26, 13.8667) measured on face at (-4.6333, 26, 13.8667) measured on face at (-4.6333, 26, 13.8667) tangent chain off on bodies 1
chamfer "Chamfer23" distance 1 distance2 1 4 edges at (14.9015, -20.6424, 10) (-17.6985, -20.6424, 10) (15.2551, 19.9111, 10) (-17.9106, 19.7697, 10) measured on face at (16.7505, -19.8831, 10) measured on face at (-16.889, -20.4401, 10) measured on face at (17.0367, 19.8916, 10) measured on face at (-16.8787, 19.6773, 10) tangent chain off on bodies 1
fillet "Fillet17" radius 2 16 edges at (-20.8142, -24.6142, 0) (-21.4, 0.4, 0) (-20.8142, 25.4142, 0) (9.4, 26, 0) (39.6142, 25.4142, 0) (40.2, 0.4, 0) (39.6142, -24.6142, 0) (9.4, -25.2, 0) (39.6142, -24.6142, 36.4) (40.2, 0.4, 36.4) (39.6142, 25.4142, 36.4) (9.4, 26, 36.4) (-20.8142, 25.4142, 36.4) (-21.4, 0.4, 36.4) (-20.8142, -24.6142, 36.4) (9.4, -25.2, 36.4) on bodies 1 2
chamfer "Chamfer20" distance 0.5 distance2 1 6 edges at (40.2, 0.4, 33.9) (40.2, 5.4, 32.65) (40.2, -4.6, 32.65) (-21.4, -4.6, 32.65) (-21.4, 0.4, 33.9) (-21.4, 5.4, 32.65) measured on face at (40.2, -17, 33.2335) measured on face at (40.2, -17, 33.2335) measured on face at (40.2, -17, 33.2335) measured on face at (-21.4, -17, 33.2335) measured on face at (-21.4, -17, 33.2335) measured on face at (-21.4, -17, 33.2335) tangent chain off on bodies 2
fillet "Fillet20" radius 2 2 edges at (22.475, -10.1404, 36.05) (-3.675, -10.1404, 36.05) on bodies 2
chamfer "Chamfer29" distance 5 distance2 1 4 edges at (9.4, 22.9, 34.4) (9.4, -22.1, 34.4) (-18.9, -22.1, 34.4) (37.7, -22.1, 34.4) measured on face at (-0.2333, 22.9, 32.4) measured on face at (0.1667, -22.1, 32.7333) measured on face at (-18.7, -22.1, 31.7333) measured on face at (37.5, -22.1, 31.7333) tangent chain off on bodies 2
chamfer "Chamfer30" distance 3 distance2 2 4 edges at (38.3, -22.7, 29.4) (38.3, 23.5, 29.4) (-19.5, 23.5, 29.4) (-19.5, -22.7, 29.4) measured on face at (18.6333, -22.9, 29.4) measured on face at (19.0333, 23.7, 29.4) measured on face at (19.0333, 23.7, 29.4) measured on face at (18.6333, -22.9, 29.4) tangent chain off on bodies 2
chamfer "Chamfer31" distance 8 angle 45 2 edges at (37.95, -10.6, 26.4) (-19.15, -17.6, 26.4) tangent chain off on bodies 2
chamfer "Chamfer32" distance 8 distance2 2.25 2 edges at (37.1, 2.9, 34.4) (-18.3, 0.4, 34.4) measured on face at (37.1, 1.0661, 31.7333) measured on face at (-18.3, -2.9339, 31.7333) tangent chain off on bodies 2
fillet "Fillet22" radius 0.4 4 edges at (38.8, 6.9, 26.4) (38.8, 5.9, 28.4) (-20, 4.4, 26.4) (-20, 3.4, 28.4) on bodies 2
fillet "Fillet23" radius 0.5 6 edges at (9.4, 24.1, 29.4) (9.4, -23.3, 29.4) (-18, -23.3, 30.4) (36.8, -23.3, 30.4) (36.8, 24.1, 30.4) (-18, 24.1, 30.4) on bodies 2
hidden bodies 1
named bodies: "Base", "Top"
